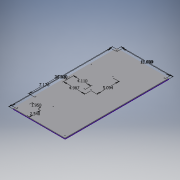
# Autodesk Inventor part: eboardbaseplate
Saved by Autodesk Inventor 2016 (Build 200138000, 138)
## iProperties
Created: 2016-01-21
Part Number: eboardbaseplate
Material: Generic
Document SubType Name: Modeling
Designer: Administrator
Density: 1 g/cm^3
Appearance: Default
Author: Administrator
Autodesk Inventor part; units mm, degrees
ref_plane "YZ Plane" through (0, 0, 0) normal (1, 0, 0) x (0, 1, 0)
ref_plane "XZ Plane" through (0, 0, 0) normal (0, 1, 0) x (-1, 0, 0)
ref_plane "XY Plane" through (0, 0, 0) normal (0, 0, 1) x (1, 0, 0)
sketch "Sketch1" plane through (0, 0, 0) normal (0, 1, 0) x (-1, 0, 0)
  line L0 (-139.7, 292.1) -> (139.7, 292.1)
  line L1 (139.7, 292.1) -> (139.7, -292.1)
  line L2 (139.7, -292.1) -> (-139.7, -292.1)
  line L3 (-139.7, -292.1) -> (-139.7, 292.1)
  line L4 (-139.7, 292.1) -> (139.7, -292.1) construction
  line L5 (139.7, 292.1) -> (-139.7, -292.1) construction
  line L6 (-152.4, 304.8) -> (152.4, 304.8)
  line L7 (152.4, 304.8) -> (152.4, -304.8)
  line L8 (152.4, -304.8) -> (-152.4, -304.8)
  line L9 (-152.4, -304.8) -> (-152.4, 304.8)
  line L10 (-152.4, 304.8) -> (152.4, -304.8) construction
  line L11 (152.4, 304.8) -> (-152.4, -304.8) construction
  line L12 (40.5945, 180.2806) -> (144.9885, 180.2806)
  line L13 (144.9885, 180.2806) -> (144.9885, -1.9898)
  line L14 (144.9885, -1.9898) -> (40.5945, -1.9898)
  line L15 (40.5945, -1.9898) -> (40.5945, 180.2806)
  line L16 (40.5945, 180.2806) -> (144.9885, -1.9898) construction
  line L17 (144.9885, 180.2806) -> (40.5945, -1.9898) construction
  line L18 (144.2829, -147.4078) -> (17.6131, -147.4078)
  line L19 (17.6131, -147.4078) -> (17.6131, -18.0202)
  line L20 (17.6131, -18.0202) -> (144.2829, -18.0202)
  line L21 (144.2829, -18.0202) -> (144.2829, -147.4078)
  line L22 (144.2829, -147.4078) -> (17.6131, -18.0202) construction
  line L23 (17.6131, -147.4078) -> (144.2829, -18.0202) construction
  line L24 (129.3166, 296.3241) -> (79.7866, 296.3241)
  line L25 (79.7866, 296.3241) -> (79.7866, 231.8081)
  line L26 (79.7866, 231.8081) -> (129.3166, 231.8081)
  line L27 (129.3166, 231.8081) -> (129.3166, 296.3241)
  line L28 (129.3166, 296.3241) -> (79.7866, 231.8081) construction
  line L29 (79.7866, 296.3241) -> (129.3166, 231.8081) construction
  point P0 (0, 0)
  point P1 (0, 0)
  point P2 (0, 0)
  point P3 (92.7915, 89.1454)
  point P4 (92.7915, 89.1454)
  point P5 (80.948, -82.714)
  point P6 (80.948, -82.714)
  point P7 (104.5516, 264.0661)
  dimension "d71" = 279.4
  dimension "d72" = 584.2
  dimension "d73" = 304.8
  dimension "d74" = 609.6
  dimension "d84" = 104.394
  dimension "d85" = 182.2704
  dimension "d86" = 126.6698
  dimension "d87" = 129.3876
  dimension "d95" = 49.53
  dimension "d96" = 64.516
  constraints: 60 end point, 14 midpoint, 12 coincident, 10 parallel, 5 horizontal, 5 perpendicular, 3 other
  measures "d71" distance of L1.end L2.end
  measures "d72" distance of L0.end L1.end
  measures "d73" distance of L7.end L8.end
  measures "d74" distance of L6.end L7.end
  measures "d84" distance of L13.end L14.end
  measures "d85" distance of L12.end L13.end
  measures "d86" distance of L19.end L20.end
  measures "d87" distance of L18.end L19.end
  measures "d95" distance of L26.end L25.end
  measures "d96" distance of L25.end L24.end
extrude "Extrusion6" add sketch "Sketch1" along normal blind 6.35 contours L0 L25 L26 L27 L1 L12 L15 L14 L20 L19 L18 L2 L3 | L25 L24 L27 L0 | L0 L27 L26 L25 | L18 L19 L20 L1 | L1 L20 L21 L18 | L12 L13 L14 L1 | L1 L14 L15 L12 | L6 L7 L8 L9
hole "Hole6" at (139.7, 0, 292.1) at (-139.7, 0, 292.1) at (-139.7, 0, -292.1) at (139.7, 0, -292.1) at (-17.6131, 0, -18.0202) at (-17.6131, 0, -147.4078) at (-144.2829, 0, -147.4078) at (-144.2829, 0, -18.0202) at (-144.9885, 0, 180.2806) at (-40.5945, 0, 180.2806) at (-40.5945, 0, -1.9898) at (-144.9885, 0, -1.9898) direction (0, 1, 0) diameter 6.35 end through all
body "Solid6"
